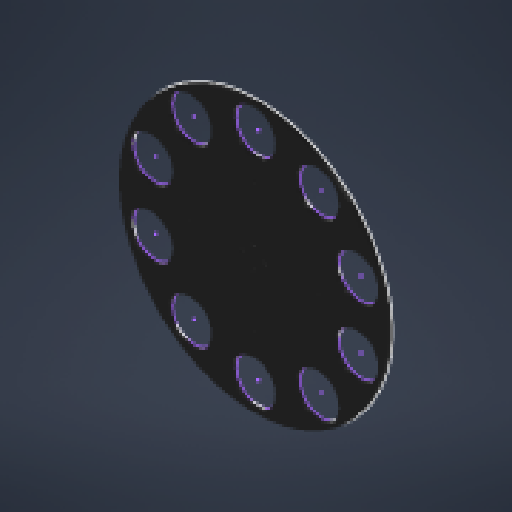
# Autodesk Inventor part: Part2
Saved by Autodesk Inventor 2027.1 (Build 311270010, 270A)
## iProperties
Created: 2026-09-28
Part Number: Part2
Material: Acetal Resin, Black
Document SubType Name: Modeling
Designer: daniel
Density: 1.425 g/cm^3
Appearance: Smooth - Black
Mass: 397.644 g
Surface Area: 1245.44 cm^2
Volume: 279.048 cm^3
Author: daniel
Autodesk Inventor part; units mm, degrees
ref_plane "YZ Plane" through (0, 0, 0) normal (1, 0, 0) x (0, 1, 0)
ref_plane "XZ Plane" through (0, 0, 0) normal (0, 1, 0) x (-1, 0, 0)
ref_plane "XY Plane" through (0, 0, 0) normal (0, 0, 1) x (1, 0, 0)
sketch "Sketch1" plane through (0, 0, 0) normal (0, 0, 1) x (1, 0, 0)
  circle A0 centre (0, 0) radius 150
  circle A1 centre (0, 0) radius 95
  circle A2 centre (0, -120) radius 25
  circle A3 centre (0, 0) radius 50
  circle A4 centre (0, 0) radius 155
  circle A5 centre (0, 0) radius 12.5
  circle A6 centre (12.5, 0) radius 2.5
  circle A7 centre (0, -12.5) radius 2.5
  circle A8 centre (-12.5, 0) radius 2.5
  circle A9 centre (0, 12.5) radius 2.5
  circle A10 centre (0, 0) radius 7
  circle A11 centre (0, 7) radius 1.6
  circle A12 centre (7, 0) radius 1.6
  circle A13 centre (0, -7) radius 1.6
  circle A14 centre (-7, 0) radius 1.6
  circle A15 centre (0, 0) radius 75
  circle A16 centre (-75, 0) radius 1.5
  circle A17 centre (0, -75) radius 1.5
  circle A18 centre (75, 0) radius 1.5
  circle A19 centre (0, 75) radius 1.5
  circle A20 centre (0, 0) radius 122.5
  circle A21 centre (-122.5, 0) radius 27.5
  circle A22 centre (-99.1046, -72.0037) radius 27.5
  circle A23 centre (-37.8546, -116.5044) radius 27.5
  circle A24 centre (37.8546, -116.5044) radius 27.5
  circle A25 centre (99.1046, -72.0037) radius 27.5
  circle A26 centre (122.5, 0) radius 27.5
  circle A27 centre (99.1046, 72.0037) radius 27.5
  circle A28 centre (37.8546, 116.5044) radius 27.5
  circle A29 centre (-37.8546, 116.5044) radius 27.5
  circle A30 centre (-99.1046, 72.0037) radius 27.5
  dimension "d36" = 150
  dimension "d42" = 245
  dimension "d0" = 300
  dimension "d1" = 190
  dimension "d2" = 50
  dimension "d7" = 100
  dimension "d13" = 310
  dimension "d17" = 25
  dimension "d18" = 5
  dimension "d19" = 5
  dimension "d20" = 5
  dimension "d21" = 5
  dimension "d29" = 14
  dimension "d30" = 3.2
  dimension "d31" = 3.2
  dimension "d32" = 3.2
  dimension "d33" = 3.2
  dimension "d37" = 3
  dimension "d40" = 360
  dimension "d43" = 55
  dimension "d46" = 360
  constraints: 29 centre point, 8 coincident, 8 point on circle, 2 horizontal alignment, 1 tangent, 34 other
  measures "d0" diameter of A0
  measures "d1" diameter of A1
  measures "d2" diameter of A2
  measures "d7" diameter of A3
  measures "d13" diameter of A4
  measures "d17" diameter of A5
  measures "d18" diameter of A6
  measures "d19" diameter of A7
  measures "d20" diameter of A8
  measures "d21" diameter of A9
  measures "d29" diameter of A10
  measures "d30" diameter of A11
  measures "d31" diameter of A12
  measures "d32" diameter of A13
  measures "d33" diameter of A14
  measures "d37" diameter of A16
  measures "d43" diameter of A21
extrude "Extrusion1" add sketch "Sketch1" along normal blind 5 contours A26 A20 A27 A0 | A0 A25 A20 A26 | A27 A20 A28 A0 | A0 A24 A20 A25 | A26 A1 A27 A20 | A20 A25 A1 A26 | A28 A20 A29 A0 | A27 A1 A28 A20 | A0 A23 A2 A24 | A20 A24 A1 A25 | A1 | A29 A20 A30 A0 | A28 A1 A29 A20 | A0 A22 A20 A23 | A2 A23 A20 A24 | A30 A20 A21 A0 | A29 A1 A30 A20 | A0 A21 A20 A22 | A20 A22 A1 A23 | A20 A23 A2 A24 | A24 A2 A1 | A30 A1 A21 A20 | A20 A21 A1 A22 | A1 A2 A23 | A3 | A4 | A6 A5 A7 A8 A9 | A10 A12 | A10 A12 | A12 A10 A13 A14 A11 | A11 A10 | A10 A11 | A13 A10 | A10 A13 | A14 A10 | A10 A14 | A18 A15 A17 A16 A19
equation "\"d0\" = 6 * Product_dia"
equation "\"d2\" = Product_dia"
equation "\"d7\" = 2 * Product_dia"
equation "\"Product_dia\" = 50"
equation "\"GridTotalSize\" = 63"
equation "\"GridBorderThickness\" = 5"
equation "\"GridBorderFillets\" = 7"
equation "\"BaseTotalWidth\" = 652"
equation "\"GridProcutClearance\" = 3"
equation "\"WorkspaceLength\" = 552"
equation "\"AxesBaseFillet\" = 15"
equation "\"WorkspaceWidth\" = 417"
equation "\"ProductTotalHeight\" = 45"
equation "\"VerticalStroke\" = 85"
equation "\"Zaxis\" = 223"
equation "\"WorkspaceHeight\" = 166.5"
equation "\"BaseTotalLength\" = 912"
equation "\"DistanceBetweenGrid\" = 5"
equation "\"CylinderStroke\" = 75"
equation "\"BaseWoodThickness\" = 7"
equation "\"kerf\" = 1.5"
equation "\"Kerf\" = 0.3"
equation "\"RxThickness\" = 1.8"
body "Solid1"
